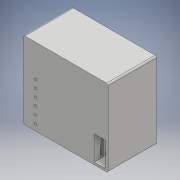
# Autodesk Inventor part: StaniceBox
Saved by Autodesk Inventor 2017 (Build 210142000, 142)
## iProperties
Created: 2019-01-28
Part Number: StaniceBox
Material: Generic
Document SubType Name: Modeling
Designer: Denis Kurka
Density: 1 g/cm^3
Appearance: Default
Author: Denis Kurka
Autodesk Inventor part; units mm, degrees
ref_plane "YZ Plane" through (0, 0, 0) normal (1, 0, 0) x (0, 1, 0)
ref_plane "XZ Plane" through (0, 0, 0) normal (0, 1, 0) x (-1, 0, 0)
ref_plane "XY Plane" through (0, 0, 0) normal (0, 0, 1) x (1, 0, 0)
sketch "Sketch1" plane through (0, 0, 0) normal (0, 1, 0) x (-1, 0, 0)
  line L0 (0, 0) -> (110, 0)
  line L1 (110, 0) -> (110, -100)
  line L2 (110, -100) -> (0, -100)
  line L3 (0, -100) -> (0, 0)
  dimension "d0" = 100
  dimension "d1" = 110
  constraints: 8 end point, 2 parallel, 1 horizontal, 1 perpendicular
  measures "d0" distance of L0.end L1.end
  measures "d1" distance of L1.end L2.end
extrude "Extrusion1" add sketch "Sketch1" along normal blind 3
sketch "Sketch2" plane through (0, 3, 0) normal (0, 1, 0) x (1, 0, 0)
  line L0 (-107, 97) -> (-3, 97)
  line L1 (-3, 97) -> (-3, 3)
  line L2 (-3, 3) -> (-107, 3)
  line L3 (-107, 3) -> (-107, 97)
  line L4 (-110, 100) -> (-110, 0) projected
  line L5 (-110, 0) -> (0, 0) projected
  line L6 (0, 0) -> (0, 100) projected
  line L7 (0, 100) -> (-110, 100) projected
  line L8 (-110, 0) -> (0, 0)
  line L9 (0, 0) -> (0, 100)
  line L10 (0, 100) -> (-110, 100)
  line L11 (-110, 100) -> (-110, 0)
  dimension "d4" = 3
  dimension "d5" = 3
  dimension "d6" = 3
  dimension "d7" = 3
  constraints: 16 end point, 4 parallel, 2 horizontal, 2 perpendicular
  measures "d4" distance between parallel lines of L4 L3
  measures "d5" distance between parallel lines of L5 L2
  measures "d6" distance between parallel lines of L6 L1
  measures "d7" distance between parallel lines of L7 L0
extrude "Extrusion2" add sketch "Sketch2" along normal blind 60
sketch "Sketch4" plane through (0, 3, 0) normal (0, 1, 0) x (1, 0, 0)
  line L0 (-107, 97) -> (-3, 97) projected
  line L1 (-102, 97) -> (-97, 97)
  line L2 (-97, 97) -> (-97, 88)
  line L3 (-97, 88) -> (-102, 88)
  line L4 (-102, 88) -> (-102, 97)
  line L5 (-91.5, 97) -> (-86.5, 97)
  line L6 (-86.5, 97) -> (-86.5, 88)
  line L7 (-86.5, 88) -> (-91.5, 88)
  line L8 (-91.5, 88) -> (-91.5, 97)
  line L9 (-102, 48) -> (-97, 48)
  line L10 (-97, 48) -> (-97, 39)
  line L11 (-97, 39) -> (-102, 39)
  line L12 (-102, 39) -> (-102, 48)
  line L13 (-91.5, 48) -> (-86.5, 48)
  line L14 (-86.5, 48) -> (-86.5, 39)
  line L15 (-86.5, 39) -> (-91.5, 39)
  line L16 (-91.5, 39) -> (-91.5, 48)
  line L17 (-107, 97) -> (-107, 3) projected
  point P0 (0, 0)
  dimension "d10" = 5
  dimension "d11" = 5.5
  dimension "d12" = 5
  dimension "d13" = 5
  dimension "d14" = 9
  dimension "d15" = 5
  dimension "d16" = 9
  dimension "d17" = 9
  dimension "d18" = 40
  constraints: 32 end point, 8 parallel, 7 point on line, 4 horizontal, 4 perpendicular
  measures "d10" distance between parallel lines of L17 L4
  measures "d11" distance between parallel lines of L2 L8
  measures "d12" distance between parallel lines of L6 L8
  measures "d13" distance between parallel lines of L4 L2
  measures "d14" distance between parallel lines of L3 L0
  measures "d15" distance between parallel lines of L14 L16
  measures "d16" distance between parallel lines of L11 L9
  measures "d17" distance between parallel lines of L15 L13
  measures "d18" distance between parallel lines of L7 L13
extrude "Extrusion3" add sketch "Sketch4" along normal blind 35
sketch "Sketch5" plane through (0, 3, 0) normal (0, 1, 0) x (1, 0, 0)
  line L0 (-102, 39) -> (-97, 39) projected
  line L1 (-102, 39) -> (-86.5, 39)
  line L2 (-86.5, 39) -> (-86.5, 36)
  line L3 (-86.5, 36) -> (-102, 36)
  line L4 (-102, 36) -> (-102, 39)
  point P0 (0, 0)
  dimension "d21" = 15.5
  dimension "d22" = 3
  constraints: 8 end point, 2 parallel, 1 horizontal, 1 perpendicular
  measures "d21" distance of L2.end L3.end
  measures "d22" distance of L3.end L0.start
extrude "Extrusion4" add sketch "Sketch5" along normal blind 5
sketch "Sketch6" plane through (0, 3, 0) normal (0, 1, 0) x (1, 0, 0)
  line L0 (-107, 97) -> (-3, 97) projected
  line L1 (-66.5, 97) -> (-50.5, 97)
  line L2 (-50.5, 97) -> (-50.5, 81)
  line L3 (-50.5, 81) -> (-66.5, 81)
  line L4 (-66.5, 81) -> (-66.5, 97)
  line L5 (-86.5, 88) -> (-86.5, 97) projected
  point P0 (0, 0)
  dimension "d25" = 16
  dimension "d26" = 16
  dimension "d27" = 20
  constraints: 8 end point, 2 parallel, 1 horizontal, 1 perpendicular, 1 point on line
  measures "d25" distance of L2.end L3.end
  measures "d26" distance of L1.end L2.end
  measures "d27" distance between parallel lines of L5 L4
extrude "Extrusion5" add sketch "Sketch6" along normal blind 5
sketch "Sketch9" plane through (-50.5, 3, -81) normal (1, 0, 0) x (0, 0, -1)
  line L0 (16, 0) -> (-78, 0) projected
  line L1 (13, 0) -> (3, 0)
  line L2 (3, 0) -> (3, 2)
  line L3 (4, 3) -> (12, 3)
  line L4 (13, 2) -> (13, 0)
  line L5 (16, 0) -> (16, 5) projected
  line L6 (0, 0) -> (0, 5) projected
  arc A0 (4, 3) -> (3, 2) centre (4, 2) ccw
  arc A1 (13, 2) -> (12, 3) centre (12, 2) ccw
  point P0 (-81, -3)
  point P1 (3, 3)
  dimension "d30" = 3
  dimension "d31" = 3
  dimension "d32" = 3
  dimension "d33" = 1
  constraints: 8 end point, 4 point on circle, 4 tangent, 3 point on line, 2 centre point, 2 parallel, 1 equal radius, 1 horizontal, 1 perpendicular
  measures "d30" distance of L1.end point (3, 3)
  measures "d31" distance between parallel lines of L5 L4
  measures "d32" distance between parallel lines of L6 L2
  measures "d33" radius of A0
extrude "Extrusion6" cut sketch "Sketch9" against normal blind 20
fillet "Fillet1" radius 1 1 edges at (-58.5, 8, -81)
fillet "Fillet2" radius 2 10 edges at (-94.25, 8, -36) (-97, 38, -43.5) (-91.5, 38, -43.5) (-102, 38, -43.5) (-86.5, 38, -43.5) (-102, 38, -92.5) (-97, 38, -92.5) (-91.5, 38, -92.5) (-86.5, 38, -92.5) (-94.25, 8, -39)
fillet "Fillet3" radius 2 8 edges at (-110, 31.5, 0) (0, 31.5, 0) (0, 31.5, -100) (-110, 31.5, -100) (-107, 33, -97) (-3, 33, -97) (-3, 33, -3) (-107, 33, -3)
fillet "Fillet4" radius 2 4 edges at (-86.5, 3, -42) (-86.5, 3, -92.5) (-102, 3, -42) (-102, 3, -92.5)
sketch "Sketch10" plane through (-86.5, 8, -39) normal (1, 0, 0) x (0, 0, -1)
  circle A0 centre (3.5, -0.75) radius 1.25
  line L0 (0, -5) -> (9, -5) projected
  line L1 (9, -5) -> (9, 28) projected
  line L2 (0, 0) -> (0, 28) projected
  circle A1 centre (3.5, 23.85) radius 1.25
  line L3 (56, -5) -> (-34, -5) projected
  line L4 (29.5, -5) -> (29.5, 28.867)
  line L5 (49, -5) -> (49, 28) projected
  circle A2 centre (55.5, -0.75) radius 1.25
  circle A3 centre (55.5, 23.85) radius 1.25
  point P0 (-39, -8)
  dimension "d41" = 4.25
  dimension "d42" = 2.5
  dimension "d43" = 5.5
  dimension "d45" = 2.5
  dimension "d46" = 24.6
  dimension "d51" = 20.5
  constraints: 4 centre point, 2 end point, 2 symmetric about line, 1 point on line, 1 vertical, 2 other
  measures "d41" distance from line of L0 A0.centre
  measures "d42" diameter of A0
  measures "d43" distance from line of L1 A0.centre
  measures "d45" diameter of A1
  measures "d46" distance of A0.centre A1.centre
  measures "d51" distance between parallel lines of L1 L4
extrude "Extrusion7" cut sketch "Sketch10" against normal blind 20
sketch "Sketch12" plane through (0, 3, 0) normal (0, 1, 0) x (1, 0, 0)
  circle A0 centre (-94.25, 92) radius 1.5
  line L0 (-91.5, 97) -> (-97, 97) projected
  line L1 (-94.25, 97) -> (-94.25, 39)
  circle A1 centre (-94.25, 82) radius 1.5
  circle A2 centre (-94.25, 72) radius 1.5
  circle A3 centre (-94.25, 62) radius 1.5
  circle A4 centre (-94.25, 52) radius 1.5
  circle A5 centre (-94.25, 42) radius 1.5
  point P0 (0, 0)
  dimension "d52" = 3
  dimension "d53" = 0
  dimension "d54" = 5
  dimension "d57" = 10
  constraints: 6 centre point, 2 end point, 2 vertical, 1 midpoint, 10 other
  measures "d52" diameter of A0
  measures "d53" distance from line of L1 A0.centre
  measures "d54" distance from line of L0 A0.centre
  measures "d57" distance of A0.centre A1.centre
extrude "Extrusion8" cut sketch "Sketch12" against normal blind 10
sketch "Sketch13" plane through (0, 3, 0) normal (0, 1, 0) x (1, 0, 0)
  line L0 (-105, 97) -> (-5, 97) projected
  line L1 (-18, 97) -> (-21, 97)
  line L2 (-21, 97) -> (-21, 62)
  line L3 (-21, 62) -> (-18, 62)
  line L4 (-18, 62) -> (-18, 97)
  line L5 (-3, 5) -> (-3, 95) projected
  line L6 (-18, 62) -> (-3, 62)
  line L7 (-3, 62) -> (-3, 65)
  line L8 (-3, 65) -> (-18, 65)
  line L9 (-18, 65) -> (-18, 62)
  point P0 (0, 0)
  dimension "d64" = 3
  dimension "d65" = 35
  dimension "d66" = 15
  dimension "d67" = 3
  constraints: 16 end point, 4 parallel, 2 horizontal, 2 perpendicular, 2 point on line
  measures "d64" distance of L2.end L3.end
  measures "d65" distance of L1.end L2.end
  measures "d66" distance between parallel lines of L5 L4
  measures "d67" distance between parallel lines of L8 L6
extrude "Extrusion9" add sketch "Sketch13" along normal blind 60
fillet "Fillet6" radius 2 3 edges at (-3, 33, -62) (-21, 33, -62) (-21, 33, -97)
sketch "Sketch14" plane through (-21, 3, -95) normal (-1, 0, 0) x (0, 0, 1)
  line L0 (29.5, 4.6993) -> (-1.5, 4.6993)
  line L1 (-1.5, 4.6993) -> (-1.5, 8.6993)
  line L2 (-1.5, 8.6993) -> (29.5, 8.6993)
  line L3 (29.5, 8.6993) -> (29.5, 4.6993)
  line L4 (-5, -3) -> (-5, 60) projected
  line L5 (33, 0) -> (33, 60) projected
  point P0 (95, -3)
  dimension "d71" = 31
  dimension "d73" = 3.5
  dimension "d74" = 4
  dimension "d75" = 3.5
  constraints: 8 end point, 2 parallel, 1 horizontal, 1 perpendicular
  measures "d71" distance of L1.end L2.end
  measures "d73" distance between parallel lines of L4 L1
  measures "d74" distance of L2.end L0.start
  measures "d75" distance between parallel lines of L5 L3
extrude "Extrusion10" cut sketch "Sketch14" along normal mid plane 10
sketch "Sketch15" plane through (-21, 3, -95) normal (-1, 0, 0) x (0, 0, 1)
  line L0 (29.5, 11.6993) -> (25.5, 11.6993)
  line L1 (25.5, 11.6993) -> (25.5, 15.6993)
  line L2 (25.5, 15.6993) -> (29.5, 15.6993)
  line L3 (29.5, 15.6993) -> (29.5, 11.6993)
  line L4 (-1.5, 11.6993) -> (2.5, 11.6993)
  line L5 (2.5, 11.6993) -> (2.5, 15.6993)
  line L6 (2.5, 15.6993) -> (-1.5, 15.6993)
  line L7 (-1.5, 15.6993) -> (-1.5, 11.6993)
  line L8 (-1.5, 8.6993) -> (-1.5, 4.6993) projected
  line L9 (29.5, 4.6993) -> (29.5, 8.6993) projected
  line L10 (29.5, 8.6993) -> (-1.5, 8.6993) projected
  point P0 (95, -3)
  dimension "d78" = 4
  dimension "d79" = 4
  dimension "d80" = 4
  dimension "d81" = 4
  dimension "d82" = 0
  dimension "d83" = 0
  dimension "d84" = 3
  constraints: 16 end point, 4 parallel, 2 horizontal, 2 perpendicular, 1 point on line
  measures "d78" distance of L1.end L2.end
  measures "d79" distance of L0.end L1.end
  measures "d80" distance of L5.end L6.end
  measures "d81" distance of L4.end L5.end
  measures "d82" distance between parallel lines of L8 L7
  measures "d83" distance between parallel lines of L9 L3
  measures "d84" distance between parallel lines of L10 L0
extrude "Extrusion11" cut sketch "Sketch15" along normal mid plane 10
fillet "Fillet7" radius 1 6 edges at (-19.8386, 18.6993, -96.5) (-19.5, 18.6993, -92.5) (-19.5, 18.6993, -69.5) (-19.5, 18.6993, -65.5) (-19.8386, 11.6993, -96.5) (-19.5, 11.6993, -65.5)
sketch "Sketch16" plane through (0, 3, 0) normal (0, 1, 0) x (1, 0, 0)
  line L0 (-3, 95) -> (-3, 65) projected
  line L1 (-18, 65) -> (-18, 97) projected
  line L2 (-3, 65) -> (-18, 65)
  line L3 (-18, 65) -> (-18, 97)
  line L4 (-18, 97) -> (-3, 97)
  line L5 (-3, 97) -> (-3, 65)
  point P0 (0, 0)
  constraints: 8 end point, 2 parallel, 1 horizontal, 1 perpendicular
extrude "Extrusion12" cut sketch "Sketch16" against normal blind 10
fillet "Fillet8" radius 2 1 edges at (-3, 1.5, -97)
sketch "Sketch17" plane through (0, 3, 0) normal (0, 1, 0) x (1, 0, 0)
  line L0 (-73, 38) -> (-3, 38)
  line L1 (-3, 38) -> (-3, 54)
  line L2 (-3, 54) -> (-73, 54)
  line L3 (-73, 54) -> (-73, 38)
  line L4 (-5, 3) -> (-105, 3) projected
  line L5 (-107, 95) -> (-107, 5) projected
  line L6 (-3, 5) -> (-3, 60) projected
  line L7 (-5, 62) -> (-19, 62) projected
  point P0 (0, 0)
  dimension "d91" = 70
  dimension "d93" = 16
  dimension "d95" = 0
  dimension "d96" = 8
  constraints: 8 end point, 2 parallel, 1 horizontal, 1 perpendicular
  measures "d91" distance of L1.end L2.end
  measures "d93" distance of L2.end L0.start
  measures "d95" distance between parallel lines of L6 L1
  measures "d96" distance between parallel lines of L7 L2
extrude "Extrusion13" add sketch "Sketch17" along normal blind 5
sketch "Sketch19" plane through (-73, 3, -38) normal (0, 0, 1) x (1, 0, 0)
  line L0 (6.5, 0) -> (-11.5, 0) projected
  line L1 (3, 0) -> (6, 0)
  line L2 (6, 0) -> (6, 3)
  line L3 (6, 3) -> (3, 3)
  line L4 (3, 3) -> (3, 0)
  line L5 (11, 0) -> (14, 0)
  line L6 (14, 0) -> (14, 3)
  line L7 (14, 3) -> (11, 3)
  line L8 (11, 3) -> (11, 0)
  line L9 (22.5, 0) -> (6.5, 0) projected
  line L10 (19, 0) -> (22, 0)
  line L11 (22, 0) -> (22, 3)
  line L12 (22, 3) -> (19, 3)
  line L13 (19, 3) -> (19, 0)
  line L14 (27, 0) -> (30, 0)
  line L15 (30, 0) -> (30, 3)
  line L16 (30, 3) -> (27, 3)
  line L17 (27, 3) -> (27, 0)
  line L18 (50, 0) -> (22.5, 0) projected
  line L19 (35, 0) -> (38, 0)
  line L20 (38, 0) -> (38, 3)
  line L21 (38, 3) -> (35, 3)
  line L22 (35, 3) -> (35, 0)
  line L23 (55, 60) -> (55, -3) projected
  line L24 (68, 0) -> (54, 0) projected
  line L25 (46, 0) -> (43, 0)
  line L26 (43, 0) -> (43, 3)
  line L27 (43, 3) -> (46, 3)
  line L28 (46, 3) -> (46, 0)
  line L29 (50, 0) -> (50, 5) projected
  point P0 (73, -3)
  dimension "d99" = 3
  dimension "d100" = 3
  dimension "d101" = 3
  dimension "d102" = 3
  dimension "d103" = 3
  dimension "d104" = 3
  dimension "d107" = 5
  dimension "d108" = 5
  dimension "d109" = 5
  dimension "d110" = 5
  dimension "d112" = 3
  dimension "d113" = 5
  dimension "d114" = 4
  constraints: 48 end point, 12 parallel, 10 point on line, 6 horizontal, 6 perpendicular
  measures "d99" distance of L3.end L1.start
  measures "d100" distance of L2.end L3.end
  measures "d101" distance of L6.end L7.end
  measures "d102" distance of L11.end L12.end
  measures "d103" distance of L15.end L16.end
  measures "d104" distance of L20.end L21.end
  measures "d107" distance between parallel lines of L2 L8
  measures "d108" distance between parallel lines of L13 L6
  measures "d109" distance between parallel lines of L17 L11
  measures "d110" distance between parallel lines of L15 L22
  measures "d112" distance of L26.end L27.end
  measures "d113" distance between parallel lines of L20 L26
  measures "d114" distance between parallel lines of L29 L28
extrude "Extrusion14" cut sketch "Sketch19" against normal blind 20
fillet "Fillet9" radius 1 12 edges at (-27, 6, -46) (-30, 6, -46) (-35, 6, -46) (-38, 6, -46) (-43, 6, -46) (-46, 6, -46) (-51, 6, -46) (-54, 6, -46) (-59, 6, -46) (-62, 6, -46) (-67, 6, -46) (-70, 6, -46)
fillet "Fillet10" radius 1 2 edges at (-73, 3, -46) (-73, 8, -46)
sketch "Sketch20" plane through (0, 3, 0) normal (0, 1, 0) x (1, 0, 0)
  line L0 (-105, 5) -> (-30, 5)
  line L1 (-30, 5) -> (-30, 30)
  line L2 (-30, 30) -> (-105, 30)
  line L3 (-105, 30) -> (-105, 5)
  line L4 (-107, 5) -> (-107, 95) projected
  line L5 (-5, 3) -> (-105, 3) projected
  point P0 (0, 0)
  dimension "d119" = 75
  dimension "d120" = 25
  dimension "d121" = 2
  dimension "d122" = 2
  constraints: 8 end point, 2 parallel, 1 horizontal, 1 perpendicular
  measures "d119" distance of L2.end L1.end
  measures "d120" distance of L0.end L1.end
  measures "d121" distance between parallel lines of L4 L3
  measures "d122" distance between parallel lines of L5 L0
extrude "Extrusion15" cut sketch "Sketch20" against normal blind 1
sketch "Sketch22" plane through (0, 3, 0) normal (0, 1, 0) x (1, 0, 0)
  line L0 (-2.8836, 5) -> (-14.8836, 5)
  line L1 (-14.8836, 5) -> (-14.8836, 25)
  line L2 (-14.8836, 25) -> (-2.8836, 25)
  line L3 (-2.8836, 25) -> (-2.8836, 5)
  line L4 (-5, 3) -> (-105, 3) projected
  point P0 (0, 0)
  dimension "d128" = 12
  dimension "d129" = 20
  dimension "d130" = 2
  constraints: 8 end point, 2 parallel, 1 horizontal, 1 perpendicular
  measures "d128" distance of L1.end L2.end
  measures "d129" distance of L0.end L1.end
  measures "d130" distance between parallel lines of L4 L0
extrude "Extrusion16" cut sketch "Sketch22" against normal blind 1
sketch "Sketch24" plane through (0, 2, 0) normal (0, 1, 0) x (1, 0, 0)
  line L0 (-14.8836, 21) -> (-8, 21)
  line L1 (-8, 21) -> (-8, 9)
  line L2 (-8, 9) -> (-14.8836, 9)
  line L3 (-14.8836, 9) -> (-14.8836, 21)
  line L4 (-3, 60) -> (-3, 5) projected
  line L5 (-14.8836, 5) -> (-14.8836, 25) projected
  line L6 (-14.8836, 25) -> (-3, 25) projected
  line L7 (-2.8836, 5) -> (-14.8836, 5) projected
  point P0 (0, 0)
  dimension "d133" = 5
  dimension "d134" = 0
  dimension "d135" = 4
  dimension "d136" = 4
  constraints: 8 end point, 2 parallel, 1 horizontal, 1 perpendicular
  measures "d133" distance between parallel lines of L4 L1
  measures "d134" distance between parallel lines of L5 L3
  measures "d135" distance between parallel lines of L6 L0
  measures "d136" distance between parallel lines of L7 L2
extrude "Extrusion17" add sketch "Sketch24" along normal blind 15 contours L0 L1 L2 L3
fillet "Fillet11" radius 1 8 edges at (-8, 9.5, -9) (-14.8836, 10, -9) (-14.8836, 10, -21) (-8, 9.5, -21) (-11.4418, 17, -21) (-14.8836, 17, -15) (-11.4418, 17, -9) (-8, 17, -15)
sketch "Sketch26" plane through (-3, 3, -54) normal (0, 0, -1) x (-1, 0, 0)
  line L0 (102, 0) -> (2, 0) projected
  line L1 (19, 0) -> (16, 0)
  line L2 (16, 0) -> (16, 2)
  line L3 (17, 3) -> (18, 3)
  line L4 (19, 2) -> (19, 0)
  line L5 (11, 0) -> (8, 0)
  line L6 (8, 0) -> (8, 2)
  line L7 (9, 3) -> (10, 3)
  line L8 (11, 2) -> (11, 0)
  line L9 (9.7968, 0) -> (6.7968, 0)
  line L10 (2, 0) -> (0, 0) projected
  line L11 (0, 0) -> (3, 0)
  line L12 (3, 0) -> (3, 2)
  line L13 (2, 3) -> (1, 3)
  line L14 (0, 2) -> (0, 0)
  line L15 (24, 2) -> (24, 0) projected
  arc A0 (1, 3) -> (0, 2) centre (1, 2) ccw
  arc A1 (3, 2) -> (2, 3) centre (2, 2) ccw
  arc A2 (9, 3) -> (8, 2) centre (9, 2) ccw
  arc A3 (11, 2) -> (10, 3) centre (10, 2) ccw
  arc A4 (17, 3) -> (16, 2) centre (17, 2) ccw
  arc A5 (19, 2) -> (18, 3) centre (18, 2) ccw
  point P0 (-3, -3)
  point P1 (16, 3)
  point P2 (19, 3)
  point P3 (8, 3)
  point P4 (11, 3)
  point P5 (3, 3)
  point P6 (0, 3)
  dimension "d140" = 3
  dimension "d141" = 3
  dimension "d143" = 3
  dimension "d144" = 3
  dimension "d146" = 5
  dimension "d147" = 3
  dimension "d148" = 5
  dimension "d149" = 5
  dimension "d150" = 1
  constraints: 26 end point, 17 point on line, 12 point on circle, 12 tangent, 6 centre point, 6 parallel, 5 equal radius, 4 horizontal, 3 perpendicular
  measures "d140" distance between parallel lines of L11 L13
  measures "d141" distance of point (3, 3) point (0, 3)
  measures "d143" distance of point (8, 3) point (11, 3)
  measures "d144" distance of point (11, 3) L5.start
  measures "d146" distance between parallel lines of L15 L4
  measures "d147" distance of point (16, 3) point (19, 3)
  measures "d148" distance between parallel lines of L2 L8
  measures "d149" distance between parallel lines of L12 L6
  measures "d150" radius of A0
extrude "Extrusion18" cut sketch "Sketch26" against normal blind 20
equation "\"d73\" = d75"
body "Solid1"
